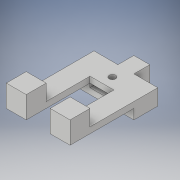
# Autodesk Inventor part: 3D Printed Y-piece
Saved by Autodesk Inventor 2018 (Build 220112000, 112)
## iProperties
Created: 2019-01-21
Part Number: 3D Printed Y-piece
Material: Generic
Document SubType Name: Modeling
Designer: maste
Density: 1 g/cm^3
Appearance: Default
Author: maste
Autodesk Inventor part; units mm, degrees
ref_plane "YZ Plane" through (0, 0, 0) normal (1, 0, 0) x (0, 1, 0)
ref_plane "XZ Plane" through (0, 0, 0) normal (0, 1, 0) x (-1, 0, 0)
ref_plane "XY Plane" through (0, 0, 0) normal (0, 0, 1) x (1, 0, 0)
sketch "Sketch1" plane through (0, 0, 0) normal (0, 0, 1) x (1, 0, 0)
  line L0 (0, 0) -> (12.7, 0)
  line L1 (12.7, 0) -> (12.7, 12.7)
  line L2 (12.7, 12.7) -> (0, 12.7)
  line L3 (0, 12.7) -> (0, 0)
  circle A0 centre (6.35, 6.35) radius 4.7625
  dimension "d0" = 12.7
  dimension "d1" = 12.7
  dimension "d2" = 9.525
  constraints: 8 end point, 2 parallel, 1 centre point, 1 horizontal, 1 perpendicular
  measures "d0" distance of L2.end L1.end
  measures "d1" distance of L1.end L0.end
  measures "d2" diameter of A0
extrude "Extrusion1" add sketch "Sketch1" along normal blind 12.7
sketch "Sketch2" plane through (0, 0, 12.7) normal (0, 0, 1) x (1, 0, 0)
  line L0 (12.7, 12.7) -> (0, 12.7) projected
  line L1 (0, 12.7) -> (-19.05, 12.7)
  line L2 (0, 12.7) -> (31.75, 12.7)
  line L3 (31.75, 12.7) -> (31.75, 0)
  line L4 (31.75, 0) -> (-19.05, 0)
  line L5 (-19.05, 0) -> (-19.05, 12.7)
  line L6 (-3.175, 7.9375) -> (15.875, 7.9375)
  line L7 (-3.175, 4.7625) -> (15.875, 4.7625)
  line L8 (15.875, 7.9375) -> (15.875, 4.7625)
  line L9 (-3.175, 7.9375) -> (-3.175, 4.7625)
  point P0 (0, 0)
  dimension "d5" = 19.05
  dimension "d6" = 31.75
  constraints: 18 end point, 3 perpendicular, 2 horizontal
  measures "d5" distance of L0.end L1.end
  measures "d6" distance of L0.end L2.end
extrude "Extrusion2" add sketch "Sketch2" along normal blind 19.05
sketch "Sketch3" plane through (0, 0, 12.7) normal (0, 0, 1) x (1, 0, 0)
  line L0 (-3.175, 7.9375) -> (15.875, 7.9375) projected
  line L1 (15.875, 4.7625) -> (-3.175, 4.7625) projected
  line L2 (-3.175, 7.9375) -> (15.875, 7.9375)
  line L3 (15.875, 7.9375) -> (15.875, 4.7625)
  line L4 (15.875, 4.7625) -> (-3.175, 4.7625)
  line L5 (-3.175, 4.7625) -> (-3.175, 7.9375)
  point P0 (0, 0)
  constraints: 8 end point, 2 parallel, 1 horizontal, 1 perpendicular
extrude "Extrusion3" add sketch "Sketch3" along normal blind 2.54
sketch "Sketch4" plane through (0, 12.7, 0) normal (0, 1, 0) x (1, 0, 0)
  line L0 (-3.175, -31.75) -> (15.875, -31.75) projected
  line L1 (6.35, -31.75) -> (6.35, -23.4188) construction
  circle A0 centre (6.35, -23.4188) radius 2.5797
  point P0 (0, 0)
  dimension "d15" = 8.3312
  dimension "d16" = 5.1594
  constraints: 2 end point, 1 centre point, 1 coincident, 1 midpoint, 1 vertical
  measures "d15" distance of L1.start L1.end
  measures "d16" diameter of A0
extrude "Extrusion4" cut sketch "Sketch4" against normal blind 20.0025
sketch "Sketch5" plane through (0, 0, 31.75) normal (0, 0, 1) x (1, 0, 0)
  line L0 (-3.175, 4.7625) -> (-3.175, 7.9375) projected
  line L1 (-19.05, 12.7) -> (-19.05, 0) projected
  line L2 (-3.175, 7.9375) -> (-19.05, 7.9375)
  line L3 (-19.05, 7.9375) -> (-19.05, 12.7)
  line L4 (-19.05, 12.7) -> (-3.175, 12.7)
  line L5 (-3.175, 12.7) -> (-3.175, 7.9375)
  line L6 (-3.175, 7.9375) -> (15.875, 7.9375) projected
  line L7 (31.75, 12.7) -> (-19.05, 12.7) projected
  line L8 (15.875, 7.9375) -> (31.75, 7.9375)
  line L9 (31.75, 7.9375) -> (31.75, 12.7)
  line L10 (31.75, 12.7) -> (15.875, 12.7)
  line L11 (15.875, 12.7) -> (15.875, 7.9375)
  point P0 (0, 0)
  constraints: 16 end point, 4 parallel, 2 horizontal, 2 perpendicular
extrude "Extrusion5" add sketch "Sketch5" along normal blind 50.8 contours L4 L5 L2 L1 | L7 L9 L8 L11
sketch "Sketch6" plane through (0, 12.7, 0) normal (0, 1, 0) x (1, 0, 0)
  line L0 (-3.175, -82.55) -> (-19.05, -82.55) projected
  line L1 (-3.175, -82.55) -> (-19.05, -82.55)
  line L2 (-19.05, -82.55) -> (-19.05, -66.675)
  line L3 (-19.05, -66.675) -> (-3.175, -66.675)
  line L4 (-3.175, -66.675) -> (-3.175, -82.55)
  line L5 (31.75, -12.7) -> (31.75, -82.55) projected
  line L6 (15.875, -31.75) -> (15.875, -82.55) projected
  line L7 (31.75, -82.55) -> (15.875, -82.55)
  line L8 (15.875, -82.55) -> (15.875, -66.675)
  line L9 (15.875, -66.675) -> (31.75, -66.675)
  line L10 (31.75, -66.675) -> (31.75, -82.55)
  point P0 (0, 0)
  dimension "d21" = 15.875
  dimension "d22" = 15.875
  constraints: 16 end point, 4 parallel, 2 horizontal, 2 perpendicular, 1 point on line
  measures "d21" distance of L2.end L3.end
  measures "d22" distance of L1.end L2.end
extrude "Extrusion6" add sketch "Sketch6" along normal blind 12.7
body "Solid1"
